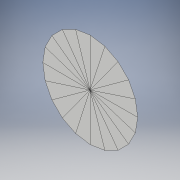
# Autodesk Inventor part: Loft1
Saved by Autodesk Inventor 2017 (Build 210142000, 142)
## iProperties
Created: 2019-01-03
Part Number: Loft1
Material: Generic
Document SubType Name: Modeling
Designer: qthuynh
Density: 1 g/cm^3
Appearance: Default
Author: qthuynh
Autodesk Inventor part; units mm, degrees
ref_plane "YZ Plane" through (0, 0, 0) normal (1, 0, 0) x (0, 1, 0)
ref_plane "XZ Plane" through (0, 0, 0) normal (0, 1, 0) x (-1, 0, 0)
sketch "Sketch1" plane through (0, 0, 0) normal (0, 0, 1) x (1, 0, 0)
  line L0 (25.4, 0) -> (25.4, 25.4)
  line L1 (25.4, 25.4) -> (0, 25.4)
  line L2 (-25.4, 0) -> (-25.4, 25.4)
  line L3 (-25.4, 25.4) -> (0, 25.4)
  line L4 (-25.4, 0) -> (-25.4, -25.4)
  line L5 (-25.4, -25.4) -> (0, -25.4)
  line L6 (25.4, 0) -> (25.4, -25.4)
  line L7 (25.4, -25.4) -> (0, -25.4)
  line L8 (25.4, -25.4) -> (-25.4, -25.4)
  line L9 (-25.4, -25.4) -> (-25.4, 25.4)
  line L10 (-25.4, 25.4) -> (25.4, 25.4)
  line L11 (25.4, 25.4) -> (25.4, -25.4)
  point P0 (0, 0)
  dimension "d0" = 25.4
  dimension "d1" = 25.4
  dimension "d2" = 25.4
  dimension "d3" = 25.4
  dimension "d4" = 25.4
  dimension "d5" = 25.4
  dimension "d6" = 25.4
  dimension "d7" = 25.4
  constraints: 24 end point, 2 parallel, 1 horizontal, 1 perpendicular
  measures "d0" distance of L1.end L0.end
  measures "d1" distance of L0.end L0.start
  measures "d2" distance of L2.end L3.end
  measures "d3" distance of L2.start L2.end
  measures "d4" distance of L5.end L4.end
  measures "d5" distance of L4.end L4.start
  measures "d6" distance of L6.end L7.end
  measures "d7" distance of L6.start L6.end
ref_plane "Work Plane2" through (0, 0, -203.2) normal (0, 0, 1) x (1, 0, 0)
ref_plane "Work Plane1" through (0, 0, -101.6) normal (0, 0, 1) x (1, 0, 0)
sketch "Sketch2" plane through (0, 0, -101.6) normal (0, 0, 1) x (1, 0, 0)
  circle A0 centre (0, 0) radius 6.35
  dimension "d10" = 12.7
  constraints: 1 centre point, 1 coincident
  measures "d10" diameter of A0
loft "Loft1" add profiles "Sketch1", "Sketch2"
sketch "Sketch4" plane through (0, 0, -203.2) normal (0, 0, 1) x (1, 0, 0)
  line L0 (0, 19711.3825) -> (6091.1522, 18746.6388)
  line L1 (6091.1522, 18746.6388) -> (11586.0599, 15946.8434)
  line L2 (11586.0599, 15946.8434) -> (15946.8434, 11586.0599)
  line L3 (15946.8434, 11586.0599) -> (18746.6388, 6091.1522)
  line L4 (18746.6388, 6091.1522) -> (19711.3825, 0)
  line L5 (19711.3825, 0) -> (18746.6388, -6091.1522)
  line L6 (18746.6388, -6091.1522) -> (15946.8434, -11586.0599)
  line L7 (15946.8434, -11586.0599) -> (11586.0599, -15946.8434)
  line L8 (11586.0599, -15946.8434) -> (6091.1522, -18746.6388)
  line L9 (6091.1522, -18746.6388) -> (0, -19711.3825)
  line L10 (0, -19711.3825) -> (-6091.1522, -18746.6388)
  line L11 (-6091.1522, -18746.6388) -> (-11586.0599, -15946.8434)
  line L12 (-11586.0599, -15946.8434) -> (-15946.8434, -11586.0599)
  line L13 (-15946.8434, -11586.0599) -> (-18746.6388, -6091.1522)
  line L14 (-18746.6388, -6091.1522) -> (-19711.3825, 0)
  line L15 (-19711.3825, 0) -> (-18746.6388, 6091.1522)
  line L16 (-18746.6388, 6091.1522) -> (-15946.8434, 11586.0599)
  line L17 (-15946.8434, 11586.0599) -> (-11586.0599, 15946.8434)
  line L18 (-11586.0599, 15946.8434) -> (-6091.1522, 18746.6388)
  line L19 (-6091.1522, 18746.6388) -> (0, 19711.3825)
  point P0 (0, 0)
  point P1 (0, 0)
  constraints: 40 end point, 1 coincident, 41 other
loft "Loft2" add profiles "Sketch4" section 1 edges at (-6.35, 0, -101.6) (0, 6.35, -101.6) (5.8666, -2.43, -101.6) (5.8666, 2.43, -101.6) (0, -6.35, -101.6)
body "Solid1"
